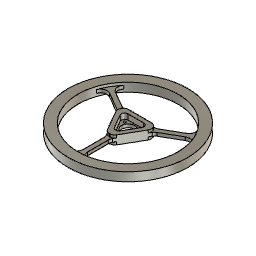
wheel (Autodesk Fusion 360 design; units mm, degrees)
Autodesk Fusion 360 part; units mm, degrees
sketch "Sketch1" plane through (0, 0, 0) normal (0, 0, 1) x (1, 0, 0)
  circle A0 centre (0, 0) radius 55
  circle A1 centre (0, 0) radius 46
  line L0 (0, -22) -> (19.0526, 11)
  line L1 (19.0526, 11) -> (-19.0526, 11)
  line L2 (-19.0526, 11) -> (0, -22)
  dimension "d3" = 110
  dimension "d4" = 92
  dimension "d33" = 22
  constraint coincident A0.centre A1.centre
  constraint concentric A0 A1
  measures "d3" diameter of A0
  measures "d4" diameter of A1
  measures "d33" distance of A0.centre L0.start
extrude "Extrude1" add sketch "Sketch1" along normal blind 8 makes body 1 at (51.7952, -2.7324, 0) makes body 2 at (0, 0, 0)
sketch "Sketch2" plane through (0, 0, 0) normal (0, 0, 1) x (1, 0, 0)
  line L0 (2, -14.0101) -> (-2, -14.0101)
  line L1 (-2, -14.0101) -> (-2, -51.9899)
  line L2 (-2, -51.9899) -> (2, -51.9899)
  line L3 (2, -51.9899) -> (2, -14.0101)
  line L4 (2, -14.0101) -> (-2, -51.9899) construction
  line L5 (-2, -14.0101) -> (2, -51.9899) construction
  point P0 (0, -33)
  point P1 (0, -33)
  dimension "d9" = 33
  dimension "d14" = 4
  dimension "d15" = 2
  constraint horizontal L0
  constraint perpendicular L0 L1
  constraint parallel L0 L2
  constraint parallel L1 L3
  constraint coincident L4 P1
  constraint coincident L5 P1
  constraint coincident P0 P1
  measures "d9" distance of origin P1
  measures "d14" distance of L0.start L0.end
  measures "d15" horizontal distance of origin L0.end
extrude "Extrude2" add sketch "Sketch2" along normal blind 8 bodies 1 2
pattern_circular "C-Pattern1" count 3 over 360 about axis through (0, 0, 1.75) along (0, 0, 1) of "Extrude2"
fillet "Fillet2" radius 6 12 edges at (17.0526, 7.5359, 4) (2, -18.5359, 4) (-40.7995, 21.2462, 4) (2, -45.9565, 4) (-15.0526, 11, 4) (15.0526, 11, 4) (38.7995, 24.7103, 4) (-2, -45.9565, 4) (-17.0526, 7.5359, 4) (-2, -18.5359, 4) (-38.7995, 24.7103, 4) (40.7995, 21.2462, 4) on bodies 1
sketch "Sketch11" plane through (0, 0, 8) normal (0, 0, 1) x (-1, 0, 0)
  line L0 (16.2487, -6.1436) -> (2.8038, 17.1436)
  arc A0 (2, 20.1436) -> (2.8038, 17.1436) centre (8, 20.1436) ccw
  line L1 (2, 20.1436) -> (2, 39.1918)
  arc A1 (9.2, 45.0706) -> (2, 39.1918) centre (8, 39.1918) ccw
  arc A2 (43.6323, -14.5679) -> (9.2, 45.0706) centre (0, 0) ccw
  arc A3 (34.9411, -17.8639) -> (43.6323, -14.5679) centre (37.9411, -12.6677) ccw
  line L2 (34.9411, -17.8639) -> (18.4449, -8.3397)
  arc A4 (16.2487, -6.1436) -> (18.4449, -8.3397) centre (21.4449, -3.1436) ccw
  line L3 (16.4449, -11.8038) -> (32.9411, -21.328)
  arc A5 (34.4323, -30.5027) -> (32.9411, -21.328) centre (29.9411, -26.5241) ccw
  arc A6 (-34.4323, -30.5027) -> (34.4323, -30.5027) centre (0, 0) ccw
  arc A7 (-32.9411, -21.328) -> (-34.4323, -30.5027) centre (-29.9411, -26.5241) ccw
  line L4 (-32.9411, -21.328) -> (-16.4449, -11.8038)
  arc A8 (-13.4449, -11) -> (-16.4449, -11.8038) centre (-13.4449, -17) ccw
  line L5 (-13.4449, -11) -> (13.4449, -11)
  arc A9 (16.4449, -11.8038) -> (13.4449, -11) centre (13.4449, -17) ccw
  arc A10 (-9.2, 45.0706) -> (-43.6323, -14.5679) centre (0, 0) ccw
  arc A11 (-2, 39.1918) -> (-9.2, 45.0706) centre (-8, 39.1918) ccw
  line L6 (-2, 39.1918) -> (-2, 20.1436)
  arc A12 (-2.8038, 17.1436) -> (-2, 20.1436) centre (-8, 20.1436) ccw
  line L7 (-2.8038, 17.1436) -> (-16.2487, -6.1436)
  arc A13 (-18.4449, -8.3397) -> (-16.2487, -6.1436) centre (-21.4449, -3.1436) ccw
  line L8 (-18.4449, -8.3397) -> (-34.9411, -17.8639)
  arc A14 (-43.6323, -14.5679) -> (-34.9411, -17.8639) centre (-37.9411, -12.6677) ccw
  circle A15 centre (0, 0) radius 55
  line L9 (0, 14.5) -> (-12.5574, -7.25)
  line L10 (-12.5574, -7.25) -> (12.5574, -7.25)
  line L11 (12.5574, -7.25) -> (0, 14.5)
  dimension "d79" = 14.5
  constraint coincident A2.centre A6.centre
  measures "d79" distance of L9.start A2.centre
extrude "Extrude7" cut sketch "Sketch11" against normal blind 5 contours L9 L10 L11 bodies 1
fillet "Fillet4" radius 3 3 edges at (12.5574, 7.25, 5.5) (-12.5574, 7.25, 5.5) (0, -14.5, 5.5) on bodies 1
sketch "Sketch12" plane through (0, 0, 3) normal (0, 0, 1) x (-1, 0, 0)
  arc A0 (2.5981, 10) -> (-2.5981, 10) centre (0, 8.5) ccw
  line L0 (-2.5981, 10) -> (-9.9593, -2.75)
  arc A1 (-9.9593, -2.75) -> (-7.3612, -7.25) centre (-7.3612, -4.25) ccw
  line L1 (-7.3612, -7.25) -> (7.3612, -7.25)
  arc A2 (7.3612, -7.25) -> (9.9593, -2.75) centre (7.3612, -4.25) ccw
  line L2 (9.9593, -2.75) -> (2.5981, 10)
  circle A3 centre (0, 0) radius 6
  dimension "d56" = 12
  constraint coincident A3.centre origin
  measures "d56" diameter of A3
extrude "Extrude8" cut sketch "Sketch12" against normal blind 3 contours A3 bodies 1
sketch "Sketch13" plane through (0, 0, 0) normal (0, 0, 1) x (1, 0, 0)
  point P0 (0, -8.5)
  dimension "d59" = 8.5
  measures "d59" distance of origin P0
hole "Hole3" at (0, -8.5, 0) direction (0, 0, 1) diameter 2.2 depth 3 tip angle 118 countersink diameter 4.5 countersink angle 90 bodies 1
pattern_circular "C-Pattern4" count 3 over 360 about axis through (0, 0, 1.75) along (0, 0, 1) of "Hole3"
sketch "Sketch14" plane through (0, 0, 8) normal (0, 0, 1) x (-1, 0, 0)
  line L0 (-9.9593, -2.75) -> (-2.5981, 10)
  arc A0 (2.5981, 10) -> (-2.5981, 10) centre (0, 8.5) ccw
  line L1 (2.5981, 10) -> (9.9593, -2.75)
  arc A1 (7.3612, -7.25) -> (9.9593, -2.75) centre (7.3612, -4.25) ccw
  line L2 (7.3612, -7.25) -> (-7.3612, -7.25)
  arc A2 (-9.9593, -2.75) -> (-7.3612, -7.25) centre (-7.3612, -4.25) ccw
  line L3 (16.2487, -6.1436) -> (2.8038, 17.1436)
  arc A3 (2, 20.1436) -> (2.8038, 17.1436) centre (8, 20.1436) ccw
  line L4 (2, 20.1436) -> (2, 39.1918)
  arc A4 (9.2, 45.0706) -> (2, 39.1918) centre (8, 39.1918) ccw
  arc A5 (43.6323, -14.5679) -> (9.2, 45.0706) centre (0, 0) ccw
  arc A6 (34.9411, -17.8639) -> (43.6323, -14.5679) centre (37.9411, -12.6677) ccw
  line L5 (34.9411, -17.8639) -> (18.4449, -8.3397)
  arc A7 (16.2487, -6.1436) -> (18.4449, -8.3397) centre (21.4449, -3.1436) ccw
  line L6 (16.4449, -11.8038) -> (32.9411, -21.328)
  arc A8 (34.4323, -30.5027) -> (32.9411, -21.328) centre (29.9411, -26.5241) ccw
  arc A9 (-34.4323, -30.5027) -> (34.4323, -30.5027) centre (0, 0) ccw
  arc A10 (-32.9411, -21.328) -> (-34.4323, -30.5027) centre (-29.9411, -26.5241) ccw
  line L7 (-32.9411, -21.328) -> (-16.4449, -11.8038)
  arc A11 (-13.4449, -11) -> (-16.4449, -11.8038) centre (-13.4449, -17) ccw
  line L8 (-13.4449, -11) -> (13.4449, -11)
  arc A12 (16.4449, -11.8038) -> (13.4449, -11) centre (13.4449, -17) ccw
  arc A13 (-9.2, 45.0706) -> (-43.6323, -14.5679) centre (0, 0) ccw
  arc A14 (-2, 39.1918) -> (-9.2, 45.0706) centre (-8, 39.1918) ccw
  line L9 (-2, 39.1918) -> (-2, 20.1436)
  arc A15 (-2.8038, 17.1436) -> (-2, 20.1436) centre (-8, 20.1436) ccw
  line L10 (-2.8038, 17.1436) -> (-16.2487, -6.1436)
  arc A16 (-18.4449, -8.3397) -> (-16.2487, -6.1436) centre (-21.4449, -3.1436) ccw
  line L11 (-18.4449, -8.3397) -> (-34.9411, -17.8639)
  arc A17 (-43.6323, -14.5679) -> (-34.9411, -17.8639) centre (-37.9411, -12.6677) ccw
  circle A18 centre (0, 0) radius 55
  circle A19 centre (0, 0) radius 46
  circle A20 centre (0, 0) radius 17
  dimension "d67" = 92
  dimension "d68" = 34
  constraint coincident A5.centre A9.centre
  measures "d67" diameter of A19
  measures "d68" diameter of A20
extrude "Extrude9" cut sketch "Sketch14" against normal blind 2.5 contours L3 A6 L5 A7 L6 A8 L8 A12 A19 A20 | L3 A3 L4 A4 A14 L9 A15 L10 A19 A20 | A10 L7 A11 L8 L10 A16 L11 A17 A19 A20 bodies 1
sketch "Sketch15" plane through (0, 0, 0) normal (0, 0, 1) x (1, 0, 0)
  circle A0 centre (0, 0) radius 46
  circle A1 centre (0, 0) radius 17
  dimension "d71" = 92
  dimension "d72" = 34
  constraint coincident A0.centre A1.centre
  constraint concentric A0 A1
  measures "d71" diameter of A0
  measures "d72" diameter of A1
extrude "Extrude10" cut sketch "Sketch15" along normal blind 2.5 bodies 1
fillet "Fillet5" radius 4.5 12 edges at (3.0455, -16.725, 6.75) (-3.0455, -16.725, 6.75) (3.0455, -16.725, 1.25) (-3.0455, -16.725, 1.25) (-16.007, 5.725, 1.25) (-12.9615, 11, 1.25) (-16.007, 5.725, 6.75) (-12.9615, 11, 6.75) (12.9615, 11, 1.25) (16.007, 5.725, 1.25) (16.007, 5.725, 6.75) (12.9615, 11, 6.75) on bodies 1
equation "diameter_inner = 92 mm"
equation "diameter_outer = 110 mm"
equation "d3 = diameter_outer"
equation "d4 = diameter_inner"
equation "thickness_outer = 8 mm"
equation "thickness_inner = thickness_outer / 2"
equation "d7 = thickness_outer"
equation "d9 = ( diameter_inner + 40 mm ) / 4"
equation "d10 = thickness_outer"
equation "diameter_shaft = 4 mm"
equation "d67 = diameter_inner"
equation "d71 = diameter_inner"
